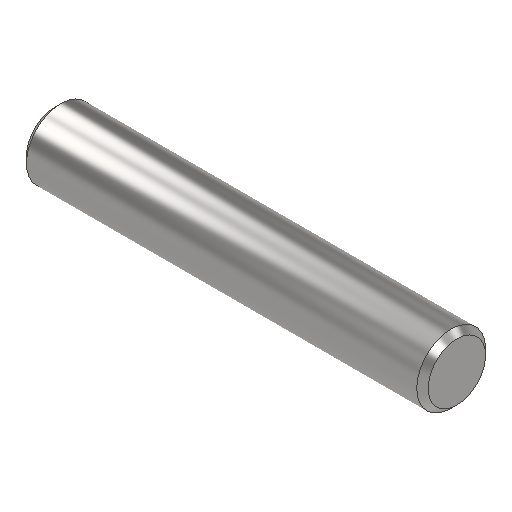
# Autodesk Inventor part: eje
Saved by Autodesk Inventor 2025.3 (Build 293356000, 356)
## iProperties
Created: 2025-11-11
Part Number: eje
Material: Stainless Steel
Document SubType Name: Modeling
Designer: Gabriel Bojaca
Density: 8 g/cm^3
Appearance: Semi-Polished
Author: Gabriel Bojaca
Autodesk Inventor part; units mm, degrees
ref_plane "YZ Plane" through (0, 0, 0) normal (1, 0, 0) x (0, 1, 0)
ref_plane "XZ Plane" through (0, 0, 0) normal (0, 1, 0) x (-1, 0, 0)
ref_plane "XY Plane" through (0, 0, 0) normal (0, 0, 1) x (1, 0, 0)
sketch "Sketch1" plane through (0, 0, 0) normal (1, 0, 0) x (0, 1, 0)
  circle A0 centre (0, 0) radius 3
  dimension "d0" = 6
  constraints: 1 centre point, 1 coincident
  measures "d0" diameter of A0
extrude "Extrusion1" add sketch "Sketch1" along normal blind 35
chamfer "Chamfer1" distance 0.5 angle 45 2 edges at (0, -3, 0) (35, -3, 0)
body "Solid1"
